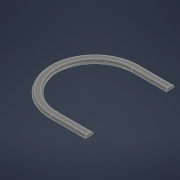
# Autodesk Inventor part: RamecekCelo
Saved by Autodesk Inventor 2022 (Build 260153000, 153)
## iProperties
Created: 2021-05-14
Part Number: RamecekCelo
Material: Generic
Document SubType Name: Modeling
Designer: jodyn
Density: 1 g/cm^3
Appearance: Gray
Author: jodyn
## iProperties of the stored document RamecekCelo_3DPrint.ipt
Created: 2021-05-14
Part Number: RamecekCelo_3DPrint
Material: Generic
Document SubType Name: Modeling
Designer: jodyn
Density: 1 g/cm^3
Appearance: Default
Author: jodyn
Autodesk Inventor part; units mm, degrees
ref_plane "YZ Plane" through (0, 0, 0) normal (1, 0, 0) x (0, 1, 0)
ref_plane "XZ Plane" through (0, 0, 0) normal (0, 1, 0) x (-1, 0, 0)
ref_plane "XY Plane" through (0, 0, 0) normal (0, 0, 1) x (1, 0, 0)
sketch "Sketch1" plane through (0, 0, 0) normal (0, 1, 0) x (-1, 0, 0)
  line L0 (85.8, 0) -> (-80.8, 0) projected
  line L1 (62, 0) -> (-57, 0)
  line L2 (0, -63) -> (0, 63)
  line L3 (0, 45) -> (-37, 45)
  line L4 (-37, -45) -> (0, -45)
  arc A0 (0, -45) -> (0, 45) centre (0, 0) ccw
  line L5 (-37, 48) -> (0, 48)
  arc A1 (0, -48) -> (0, 48) centre (0, 0) ccw
  line L6 (0, -48) -> (-37, -48)
  line L7 (-37, 48) -> (-37, 45)
  line L8 (-37, -45) -> (-37, -48)
  dimension "d7" = 3
  constraints: 16 end point, 5 point on line, 4 point on circle, 2 centre point, 2 parallel, 1 horizontal, 1 midpoint, 1 perpendicular, 1 other
  measures "d7" distance between parallel lines of L3 L5
extrude "Extrusion1" add sketch "Sketch1" along normal blind 3 contours A1 L2 A0 L0 | L0 A0 L2 A1 | L6 L8 L4 L2 | L2 L3 L7 L5
sketch "Sketch2" plane through (0, 3, 0) normal (0, 1, 0) x (1, 0, 0)
  line L0 (0, -42) -> (40, -42)
  line L1 (40, -51) -> (0, -51)
  arc A0 (0, 51) -> (0, -51) centre (0, 0) ccw
  line L2 (0, 51) -> (40, 51)
  line L3 (40, 42) -> (0, 42)
  arc A1 (0, 42) -> (0, -42) centre (0, 0) ccw
  line L4 (37, -45) -> (0, -45) projected
  line L5 (40, -51) -> (40, -42)
  line L6 (40, 42) -> (40, 51)
  point P0 (43, -45)
  point P1 (40, -45)
  constraints: 12 end point, 4 point on circle, 3 point on line, 2 centre point, 1 perpendicular
extrude "Extrusion2" add sketch "Sketch2" along normal blind 3
fillet "Fillet1" radius 2 6 edges at (20, 6, 51) (20, 6, 42) (-42, 6, 0) (20, 6, -42) (20, 6, -51) (-51, 6, 0)
body "Solid1"
